Autodesk Fusion 360 part; units mm, degrees
(part 2 of 3)
  spline S18 degree 5 poles (-8.9859, 5.2547) (-8.9893, 5.2567) (-8.9962, 5.2606) (-9.0067, 5.2662) (-9.0209, 5.2733) (-9.0389, 5.2815) (-9.0573, 5.2892) (-9.0757, 5.2967) (-9.0943, 5.304) (-9.1129, 5.3112) (-9.1316, 5.3183) (-9.1504, 5.3252) (-9.1692, 5.332) (-9.1882, 5.3385) (-9.2073, 5.3449) (-9.2265, 5.351) (-9.2458, 5.3569) (-9.2651, 5.3627) (-9.2846, 5.3684) (-9.3041, 5.3739) (-9.3236, 5.3793) (-9.3432, 5.3846) (-9.3629, 5.3898) (-9.3827, 5.3948) (-9.4025, 5.3997) (-9.4224, 5.4044) (-9.4423, 5.409) (-9.4623, 5.4135) (-9.4824, 5.4179) (-9.5025, 5.4221) (-9.5226, 5.4263) (-9.5429, 5.4303) (-9.5631, 5.4342) (-9.5835, 5.438) (-9.6038, 5.4417) (-9.6242, 5.4453) (-9.6447, 5.4488) (-9.6652, 5.4521) (-9.6858, 5.4554) (-9.7064, 5.4585) (-9.7271, 5.4616) (-9.7478, 5.4645) (-9.7685, 5.4674) (-9.7893, 5.4701) (-9.8101, 5.4727) (-9.831, 5.4753) (-9.8519, 5.4777) (-9.8729, 5.4801) (-9.8939, 5.4823) (-9.9149, 5.4844) (-9.936, 5.4865) (-9.9571, 5.4884) (-9.9783, 5.4903) (-9.9994, 5.4921) (-10.0207, 5.4937) (-10.0419, 5.4953) (-10.0632, 5.4968) (-10.0845, 5.4982) (-10.1059, 5.4995) (-10.1273, 5.5007) (-10.1487, 5.5018) (-10.1702, 5.5028) (-10.1917, 5.5037) (-10.2132, 5.5046) (-10.2348, 5.5053) (-10.2564, 5.506) (-10.278, 5.5066) (-10.2997, 5.507) (-10.3213, 5.5074) (-10.3431, 5.5078) (-10.3648, 5.508) (-10.3822, 5.5081) (-10.3953, 5.5081) (-10.404, 5.5081) (-10.4084, 5.5081) knots 0 0 0 0 0 0 0.01428571 0.02857143 0.04285714 0.05714286 0.07142857 0.08571429 0.1 0.11428571 0.12857143 0.14285714 0.15714286 0.17142857 0.18571429 0.2 0.21428571 0.22857143 0.24285714 0.25714286 0.27142857 0.28571429 0.3 0.31428571 0.32857143 0.34285714 0.35714286 0.37142857 0.38571429 0.4 0.41428571 0.42857143 0.44285714 0.45714286 0.47142857 0.48571429 0.5 0.51428571 0.52857143 0.54285714 0.55714286 0.57142857 0.58571429 0.6 0.61428571 0.62857143 0.64285714 0.65714286 0.67142857 0.68571429 0.7 0.71428571 0.72857143 0.74285714 0.75714286 0.77142857 0.78571429 0.8 0.81428571 0.82857143 0.84285714 0.85714286 0.87142857 0.88571429 0.9 0.91428571 0.92857143 0.94285714 0.95714286 0.97142857 0.98571429 1 1 1 1 1 1
  arc A38 (-10.4084, 5.5081) -> (-10.796, 4.7033) centre (0, 0) ccw
  spline S19 degree 5 poles (-10.796, 4.7033) (-10.7932, 4.6999) (-10.7878, 4.6931) (-10.7796, 4.6829) (-10.7687, 4.6694) (-10.7549, 4.6525) (-10.7411, 4.6357) (-10.7273, 4.619) (-10.7134, 4.6024) (-10.6995, 4.5858) (-10.6855, 4.5694) (-10.6715, 4.553) (-10.6574, 4.5367) (-10.6433, 4.5204) (-10.6291, 4.5043) (-10.6149, 4.4882) (-10.6006, 4.4723) (-10.5863, 4.4564) (-10.5719, 4.4405) (-10.5574, 4.4248) (-10.543, 4.4092) (-10.5284, 4.3936) (-10.5138, 4.3782) (-10.4992, 4.3628) (-10.4845, 4.3475) (-10.4698, 4.3323) (-10.455, 4.3172) (-10.4401, 4.3022) (-10.4252, 4.2873) (-10.4103, 4.2724) (-10.3953, 4.2577) (-10.3802, 4.243) (-10.3651, 4.2285) (-10.35, 4.214) (-10.3348, 4.1997) (-10.3195, 4.1854) (-10.3042, 4.1713) (-10.2888, 4.1572) (-10.2734, 4.1433) (-10.2579, 4.1295) (-10.2424, 4.1157) (-10.2268, 4.1021) (-10.2112, 4.0886) (-10.1955, 4.0752) (-10.1797, 4.0619) (-10.1639, 4.0487) (-10.148, 4.0356) (-10.1321, 4.0227) (-10.1161, 4.0098) (-10.1001, 3.9971) (-10.084, 3.9845) (-10.0678, 3.9721) (-10.0516, 3.9597) (-10.0353, 3.9476) (-10.0189, 3.9355) (-10.0025, 3.9236) (-9.986, 3.9118) (-9.9694, 3.9002) (-9.9529, 3.8886) (-9.9362, 3.8773) (-9.9194, 3.8661) (-9.9026, 3.8551) (-9.8856, 3.8444) (-9.8686, 3.8338) (-9.8514, 3.8235) (-9.8342, 3.8133) (-9.817, 3.8032) (-9.7997, 3.7933) (-9.7824, 3.7835) (-9.7649, 3.774) (-9.7472, 3.765) (-9.7329, 3.7583) (-9.7219, 3.7536) (-9.7146, 3.7507) (-9.7109, 3.7492) knots -1 -1 -1 -1 -1 -1 -0.98571429 -0.97142857 -0.95714286 -0.94285714 -0.92857143 -0.91428571 -0.9 -0.88571429 -0.87142857 -0.85714286 -0.84285714 -0.82857143 -0.81428571 -0.8 -0.78571429 -0.77142857 -0.75714286 -0.74285714 -0.72857143 -0.71428571 -0.7 -0.68571429 -0.67142857 -0.65714286 -0.64285714 -0.62857143 -0.61428571 -0.6 -0.58571429 -0.57142857 -0.55714286 -0.54285714 -0.52857143 -0.51428571 -0.5 -0.48571429 -0.47142857 -0.45714286 -0.44285714 -0.42857143 -0.41428571 -0.4 -0.38571429 -0.37142857 -0.35714286 -0.34285714 -0.32857143 -0.31428571 -0.3 -0.28571429 -0.27142857 -0.25714286 -0.24285714 -0.22857143 -0.21428571 -0.2 -0.18571429 -0.17142857 -0.15714286 -0.14285714 -0.12857143 -0.11428571 -0.1 -0.08571429 -0.07142857 -0.05714286 -0.04285714 -0.02857143 -0.01428571 0 0 0 0 0 0
  line L19 (-9.7109, 3.7492) -> (-9.3969, 3.6277)
  arc A39 (-9.0296, 2.8622) -> (-9.3969, 3.6277) centre (-9.6207, 3.0495) ccw
  arc A40 (-9.0296, 2.8622) -> (-9.0729, 2.7218) centre (0, 0) ccw
  arc A41 (-9.8076, 2.2961) -> (-9.0729, 2.7218) centre (-9.6668, 2.8999) ccw
  line L20 (-9.8076, 2.2961) -> (-10.1355, 2.3726)
  spline S20 degree 5 poles (-10.1355, 2.3726) (-10.1394, 2.3735) (-10.1471, 2.3752) (-10.1588, 2.3775) (-10.1744, 2.38) (-10.1941, 2.3826) (-10.2139, 2.3846) (-10.2337, 2.3862) (-10.2536, 2.3877) (-10.2736, 2.3891) (-10.2935, 2.3904) (-10.3135, 2.3915) (-10.3335, 2.3924) (-10.3536, 2.3931) (-10.3737, 2.3935) (-10.3938, 2.3937) (-10.414, 2.3937) (-10.4342, 2.3935) (-10.4544, 2.3932) (-10.4747, 2.3927) (-10.495, 2.3922) (-10.5153, 2.3914) (-10.5356, 2.3905) (-10.5559, 2.3895) (-10.5763, 2.3883) (-10.5967, 2.387) (-10.6171, 2.3855) (-10.6376, 2.3839) (-10.658, 2.3822) (-10.6785, 2.3803) (-10.699, 2.3784) (-10.7195, 2.3762) (-10.74, 2.374) (-10.7606, 2.3717) (-10.7811, 2.3692) (-10.8017, 2.3666) (-10.8223, 2.3639) (-10.8429, 2.361) (-10.8635, 2.3581) (-10.8841, 2.355) (-10.9048, 2.3518) (-10.9254, 2.3485) (-10.9461, 2.3451) (-10.9667, 2.3416) (-10.9874, 2.338) (-11.0081, 2.3343) (-11.0288, 2.3304) (-11.0495, 2.3265) (-11.0703, 2.3225) (-11.091, 2.3183) (-11.1117, 2.3141) (-11.1325, 2.3097) (-11.1532, 2.3052) (-11.174, 2.3007) (-11.1948, 2.296) (-11.2156, 2.2913) (-11.2363, 2.2864) (-11.2571, 2.2814) (-11.2779, 2.2764) (-11.2987, 2.2712) (-11.3195, 2.266) (-11.3403, 2.2606) (-11.3612, 2.2552) (-11.382, 2.2496) (-11.4028, 2.244) (-11.4236, 2.2382) (-11.4445, 2.2324) (-11.4653, 2.2265) (-11.4861, 2.2205) (-11.507, 2.2144) (-11.5278, 2.2082) (-11.5445, 2.2032) (-11.557, 2.1993) (-11.5654, 2.1968) (-11.5695, 2.1955) knots 0 0 0 0 0 0 0.01428571 0.02857143 0.04285714 0.05714286 0.07142857 0.08571429 0.1 0.11428571 0.12857143 0.14285714 0.15714286 0.17142857 0.18571429 0.2 0.21428571 0.22857143 0.24285714 0.25714286 0.27142857 0.28571429 0.3 0.31428571 0.32857143 0.34285714 0.35714286 0.37142857 0.38571429 0.4 0.41428571 0.42857143 0.44285714 0.45714286 0.47142857 0.48571429 0.5 0.51428571 0.52857143 0.54285714 0.55714286 0.57142857 0.58571429 0.6 0.61428571 0.62857143 0.64285714 0.65714286 0.67142857 0.68571429 0.7 0.71428571 0.72857143 0.74285714 0.75714286 0.77142857 0.78571429 0.8 0.81428571 0.82857143 0.84285714 0.85714286 0.87142857 0.88571429 0.9 0.91428571 0.92857143 0.94285714 0.95714286 0.97142857 0.98571429 1 1 1 1 1 1
  arc A42 (-11.5695, 2.1955) -> (-11.7027, 1.3122) centre (0, 0) ccw
  spline S21 degree 5 poles (-11.7027, 1.3122) (-11.6991, 1.3098) (-11.6918, 1.3049) (-11.681, 1.2975) (-11.6666, 1.2878) (-11.6485, 1.2757) (-11.6304, 1.2638) (-11.6122, 1.2519) (-11.594, 1.2401) (-11.5759, 1.2284) (-11.5576, 1.2168) (-11.5394, 1.2052) (-11.5211, 1.1938) (-11.5029, 1.1824) (-11.4845, 1.1712) (-11.4662, 1.16) (-11.4479, 1.149) (-11.4295, 1.138) (-11.4111, 1.1272) (-11.3926, 1.1164) (-11.3742, 1.1057) (-11.3557, 1.0951) (-11.3372, 1.0847) (-11.3187, 1.0743) (-11.3002, 1.064) (-11.2816, 1.0538) (-11.263, 1.0437) (-11.2444, 1.0338) (-11.2258, 1.0239) (-11.2071, 1.0141) (-11.1884, 1.0045) (-11.1697, 0.9949) (-11.151, 0.9855) (-11.1323, 0.9761) (-11.1135, 0.9669) (-11.0947, 0.9578) (-11.0759, 0.9488) (-11.0571, 0.9399) (-11.0382, 0.9311) (-11.0194, 0.9224) (-11.0005, 0.9139) (-10.9816, 0.9054) (-10.9626, 0.8971) (-10.9437, 0.889) (-10.9247, 0.8809) (-10.9057, 0.873) (-10.8867, 0.8652) (-10.8677, 0.8575) (-10.8486, 0.8499) (-10.8295, 0.8425) (-10.8104, 0.8352) (-10.7913, 0.8281) (-10.7722, 0.8211) (-10.753, 0.8142) (-10.7338, 0.8076) (-10.7146, 0.801) (-10.6954, 0.7946) (-10.6761, 0.7884) (-10.6569, 0.7822) (-10.6376, 0.7763) (-10.6183, 0.7705) (-10.5989, 0.765) (-10.5796, 0.7597) (-10.5602, 0.7547) (-10.5408, 0.7499) (-10.5213, 0.7452) (-10.5019, 0.7407) (-10.4824, 0.7362) (-10.463, 0.732) (-10.4435, 0.7281) (-10.4239, 0.7247) (-10.4082, 0.7225) (-10.3964, 0.7213) (-10.3885, 0.7206) (-10.3846, 0.7203) knots -1 -1 -1 -1 -1 -1 -0.98571429 -0.97142857 -0.95714286 -0.94285714 -0.92857143 -0.91428571 -0.9 -0.88571429 -0.87142857 -0.85714286 -0.84285714 -0.82857143 -0.81428571 -0.8 -0.78571429 -0.77142857 -0.75714286 -0.74285714 -0.72857143 -0.71428571 -0.7 -0.68571429 -0.67142857 -0.65714286 -0.64285714 -0.62857143 -0.61428571 -0.6 -0.58571429 -0.57142857 -0.55714286 -0.54285714 -0.52857143 -0.51428571 -0.5 -0.48571429 -0.47142857 -0.45714286 -0.44285714 -0.42857143 -0.41428571 -0.4 -0.38571429 -0.37142857 -0.35714286 -0.34285714 -0.32857143 -0.31428571 -0.3 -0.28571429 -0.27142857 -0.25714286 -0.24285714 -0.22857143 -0.21428571 -0.2 -0.18571429 -0.17142857 -0.15714286 -0.14285714 -0.12857143 -0.11428571 -0.1 -0.08571429 -0.07142857 -0.05714286 -0.04285714 -0.02857143 -0.01428571 0 0 0 0 0 0
  line L21 (-10.3846, 0.7203) -> (-10.0487, 0.6968)
  arc A43 (-9.4721, 0.0735) -> (-10.0487, 0.6968) centre (-10.0921, 0.0783) ccw
  arc A44 (-9.4721, 0.0735) -> (-9.4721, -0.0735) centre (0, 0) ccw
  arc A45 (-10.0487, -0.6968) -> (-9.4721, -0.0735) centre (-10.0921, -0.0783) ccw
  line L22 (-10.0487, -0.6968) -> (-10.3846, -0.7203)
  spline S22 degree 5 poles (-10.3846, -0.7203) (-10.3885, -0.7206) (-10.3964, -0.7213) (-10.4082, -0.7225) (-10.4239, -0.7247) (-10.4435, -0.7281) (-10.463, -0.732) (-10.4824, -0.7362) (-10.5019, -0.7407) (-10.5213, -0.7452) (-10.5408, -0.7499) (-10.5602, -0.7547) (-10.5796, -0.7597) (-10.5989, -0.765) (-10.6183, -0.7705) (-10.6376, -0.7763) (-10.6569, -0.7822) (-10.6761, -0.7884) (-10.6954, -0.7946) (-10.7146, -0.801) (-10.7338, -0.8076) (-10.753, -0.8142) (-10.7722, -0.8211) (-10.7913, -0.8281) (-10.8104, -0.8352) (-10.8295, -0.8425) (-10.8486, -0.8499) (-10.8677, -0.8575) (-10.8867, -0.8652) (-10.9057, -0.873) (-10.9247, -0.8809) (-10.9437, -0.889) (-10.9626, -0.8971) (-10.9816, -0.9054) (-11.0005, -0.9139) (-11.0194, -0.9224) (-11.0382, -0.9311) (-11.0571, -0.9399) (-11.0759, -0.9488) (-11.0947, -0.9578) (-11.1135, -0.9669) (-11.1323, -0.9761) (-11.151, -0.9855) (-11.1697, -0.9949) (-11.1884, -1.0045) (-11.2071, -1.0141) (-11.2258, -1.0239) (-11.2444, -1.0338) (-11.263, -1.0437) (-11.2816, -1.0538) (-11.3002, -1.064) (-11.3187, -1.0743) (-11.3372, -1.0847) (-11.3557, -1.0951) (-11.3742, -1.1057) (-11.3926, -1.1164) (-11.4111, -1.1272) (-11.4295, -1.138) (-11.4479, -1.149) (-11.4662, -1.16) (-11.4845, -1.1712) (-11.5029, -1.1824) (-11.5211, -1.1938) (-11.5394, -1.2052) (-11.5576, -1.2168) (-11.5759, -1.2284) (-11.594, -1.2401) (-11.6122, -1.2519) (-11.6304, -1.2638) (-11.6485, -1.2757) (-11.6666, -1.2878) (-11.681, -1.2975) (-11.6918, -1.3049) (-11.6991, -1.3098) (-11.7027, -1.3122) knots 0 0 0 0 0 0 0.01428571 0.02857143 0.04285714 0.05714286 0.07142857 0.08571429 0.1 0.11428571 0.12857143 0.14285714 0.15714286 0.17142857 0.18571429 0.2 0.21428571 0.22857143 0.24285714 0.25714286 0.27142857 0.28571429 0.3 0.31428571 0.32857143 0.34285714 0.35714286 0.37142857 0.38571429 0.4 0.41428571 0.42857143 0.44285714 0.45714286 0.47142857 0.48571429 0.5 0.51428571 0.52857143 0.54285714 0.55714286 0.57142857 0.58571429 0.6 0.61428571 0.62857143 0.64285714 0.65714286 0.67142857 0.68571429 0.7 0.71428571 0.72857143 0.74285714 0.75714286 0.77142857 0.78571429 0.8 0.81428571 0.82857143 0.84285714 0.85714286 0.87142857 0.88571429 0.9 0.91428571 0.92857143 0.94285714 0.95714286 0.97142857 0.98571429 1 1 1 1 1 1
  arc A46 (-11.7027, -1.3122) -> (-11.5695, -2.1955) centre (0, 0) ccw
  spline S23 degree 5 poles (-11.5695, -2.1955) (-11.5654, -2.1968) (-11.557, -2.1993) (-11.5445, -2.2032) (-11.5278, -2.2082) (-11.507, -2.2144) (-11.4861, -2.2205) (-11.4653, -2.2265) (-11.4445, -2.2324) (-11.4236, -2.2382) (-11.4028, -2.244) (-11.382, -2.2496) (-11.3612, -2.2552) (-11.3403, -2.2606) (-11.3195, -2.266) (-11.2987, -2.2712) (-11.2779, -2.2764) (-11.2571, -2.2814) (-11.2363, -2.2864) (-11.2156, -2.2913) (-11.1948, -2.296) (-11.174, -2.3007) (-11.1532, -2.3052) (-11.1325, -2.3097) (-11.1117, -2.3141) (-11.091, -2.3183) (-11.0703, -2.3225) (-11.0495, -2.3265) (-11.0288, -2.3304) (-11.0081, -2.3343) (-10.9874, -2.338) (-10.9667, -2.3416) (-10.9461, -2.3451) (-10.9254, -2.3485) (-10.9048, -2.3518) (-10.8841, -2.355) (-10.8635, -2.3581) (-10.8429, -2.361) (-10.8223, -2.3639) (-10.8017, -2.3666) (-10.7811, -2.3692) (-10.7606, -2.3717) (-10.74, -2.374) (-10.7195, -2.3762) (-10.699, -2.3784) (-10.6785, -2.3803) (-10.658, -2.3822) (-10.6376, -2.3839) (-10.6171, -2.3855) (-10.5967, -2.387) (-10.5763, -2.3883) (-10.5559, -2.3895) (-10.5356, -2.3905) (-10.5153, -2.3914) (-10.495, -2.3922) (-10.4747, -2.3927) (-10.4544, -2.3932) (-10.4342, -2.3935) (-10.414, -2.3937) (-10.3938, -2.3937) (-10.3737, -2.3935) (-10.3536, -2.3931) (-10.3335, -2.3924) (-10.3135, -2.3915) (-10.2935, -2.3904) (-10.2736, -2.3891) (-10.2536, -2.3877) (-10.2337, -2.3862) (-10.2139, -2.3846) (-10.1941, -2.3826) (-10.1744, -2.38) (-10.1588, -2.3775) (-10.1471, -2.3752) (-10.1394, -2.3735) (-10.1355, -2.3726) knots -1 -1 -1 -1 -1 -1 -0.98571429 -0.97142857 -0.95714286 -0.94285714 -0.92857143 -0.91428571 -0.9 -0.88571429 -0.87142857 -0.85714286 -0.84285714 -0.82857143 -0.81428571 -0.8 -0.78571429 -0.77142857 -0.75714286 -0.74285714 -0.72857143 -0.71428571 -0.7 -0.68571429 -0.67142857 -0.65714286 -0.64285714 -0.62857143 -0.61428571 -0.6 -0.58571429 -0.57142857 -0.55714286 -0.54285714 -0.52857143 -0.51428571 -0.5 -0.48571429 -0.47142857 -0.45714286 -0.44285714 -0.42857143 -0.41428571 -0.4 -0.38571429 -0.37142857 -0.35714286 -0.34285714 -0.32857143 -0.31428571 -0.3 -0.28571429 -0.27142857 -0.25714286 -0.24285714 -0.22857143 -0.21428571 -0.2 -0.18571429 -0.17142857 -0.15714286 -0.14285714 -0.12857143 -0.11428571 -0.1 -0.08571429 -0.07142857 -0.05714286 -0.04285714 -0.02857143 -0.01428571 0 0 0 0 0 0
  line L23 (-10.1355, -2.3726) -> (-9.8076, -2.2961)
  arc A47 (-9.0729, -2.7218) -> (-9.8076, -2.2961) centre (-9.6668, -2.8999) ccw
  arc A48 (-9.0729, -2.7218) -> (-9.0296, -2.8622) centre (0, 0) ccw
  arc A49 (-9.3969, -3.6277) -> (-9.0296, -2.8622) centre (-9.6207, -3.0495) ccw
  line L24 (-9.3969, -3.6277) -> (-9.7109, -3.7492)
  spline S24 degree 5 poles (-9.7109, -3.7492) (-9.7146, -3.7507) (-9.7219, -3.7536) (-9.7329, -3.7583) (-9.7472, -3.765) (-9.7649, -3.774) (-9.7824, -3.7835) (-9.7997, -3.7933) (-9.817, -3.8032) (-9.8342, -3.8133) (-9.8514, -3.8235) (-9.8686, -3.8338) (-9.8856, -3.8444) (-9.9026, -3.8551) (-9.9194, -3.8661) (-9.9362, -3.8773) (-9.9529, -3.8886) (-9.9694, -3.9002) (-9.986, -3.9118) (-10.0025, -3.9236) (-10.0189, -3.9355) (-10.0353, -3.9476) (-10.0516, -3.9597) (-10.0678, -3.9721) (-10.084, -3.9845) (-10.1001, -3.9971) (-10.1161, -4.0098) (-10.1321, -4.0227) (-10.148, -4.0356) (-10.1639, -4.0487) (-10.1797, -4.0619) (-10.1955, -4.0752) (-10.2112, -4.0886) (-10.2268, -4.1021) (-10.2424, -4.1157) (-10.2579, -4.1295) (-10.2734, -4.1433) (-10.2888, -4.1572) (-10.3042, -4.1713) (-10.3195, -4.1854) (-10.3348, -4.1997) (-10.35, -4.214) (-10.3651, -4.2285) (-10.3802, -4.243) (-10.3953, -4.2577) (-10.4103, -4.2724) (-10.4252, -4.2873) (-10.4401, -4.3022) (-10.455, -4.3172) (-10.4698, -4.3323) (-10.4845, -4.3475) (-10.4992, -4.3628) (-10.5138, -4.3782) (-10.5284, -4.3936) (-10.543, -4.4092) (-10.5574, -4.4248) (-10.5719, -4.4405) (-10.5863, -4.4564) (-10.6006, -4.4723) (-10.6149, -4.4882) (-10.6291, -4.5043) (-10.6433, -4.5204) (-10.6574, -4.5367) (-10.6715, -4.553) (-10.6855, -4.5694) (-10.6995, -4.5858) (-10.7134, -4.6024) (-10.7273, -4.619) (-10.7411, -4.6357) (-10.7549, -4.6525) (-10.7687, -4.6694) (-10.7796, -4.6829) (-10.7878, -4.6931) (-10.7932, -4.6999) (-10.796, -4.7033) knots 0 0 0 0 0 0 0.01428571 0.02857143 0.04285714 0.05714286 0.07142857 0.08571429 0.1 0.11428571 0.12857143 0.14285714 0.15714286 0.17142857 0.18571429 0.2 0.21428571 0.22857143 0.24285714 0.25714286 0.27142857 0.28571429 0.3 0.31428571 0.32857143 0.34285714 0.35714286 0.37142857 0.38571429 0.4 0.41428571 0.42857143 0.44285714 0.45714286 0.47142857 0.48571429 0.5 0.51428571 0.52857143 0.54285714 0.55714286 0.57142857 0.58571429 0.6 0.61428571 0.62857143 0.64285714 0.65714286 0.67142857 0.68571429 0.7 0.71428571 0.72857143 0.74285714 0.75714286 0.77142857 0.78571429 0.8 0.81428571 0.82857143 0.84285714 0.85714286 0.87142857 0.88571429 0.9 0.91428571 0.92857143 0.94285714 0.95714286 0.97142857 0.98571429 1 1 1 1 1 1
  arc A50 (-10.796, -4.7033) -> (-10.4084, -5.5081) centre (0, 0) ccw
  spline S25 degree 5 poles (-10.4084, -5.5081) (-10.404, -5.5081) (-10.3953, -5.5081) (-10.3822, -5.5081) (-10.3648, -5.508) (-10.3431, -5.5078) (-10.3213, -5.5074) (-10.2997, -5.507) (-10.278, -5.5066) (-10.2564, -5.506) (-10.2348, -5.5053) (-10.2132, -5.5046) (-10.1917, -5.5037) (-10.1702, -5.5028) (-10.1487, -5.5018) (-10.1273, -5.5007) (-10.1059, -5.4995) (-10.0845, -5.4982) (-10.0632, -5.4968) (-10.0419, -5.4953) (-10.0207, -5.4937) (-9.9994, -5.4921) (-9.9783, -5.4903) (-9.9571, -5.4884) (-9.936, -5.4865) (-9.9149, -5.4844) (-9.8939, -5.4823) (-9.8729, -5.4801) (-9.8519, -5.4777) (-9.831, -5.4753) (-9.8101, -5.4727) (-9.7893, -5.4701) (-9.7685, -5.4674) (-9.7478, -5.4645) (-9.7271, -5.4616) (-9.7064, -5.4585) (-9.6858, -5.4554) (-9.6652, -5.4521) (-9.6447, -5.4488) (-9.6242, -5.4453) (-9.6038, -5.4417) (-9.5835, -5.438) (-9.5631, -5.4342) (-9.5429, -5.4303) (-9.5226, -5.4263) (-9.5025, -5.4221) (-9.4824, -5.4179) (-9.4623, -5.4135) (-9.4423, -5.409) (-9.4224, -5.4044) (-9.4025, -5.3997) (-9.3827, -5.3948) (-9.3629, -5.3898) (-9.3432, -5.3846) (-9.3236, -5.3793) (-9.3041, -5.3739) (-9.2846, -5.3684) (-9.2651, -5.3627) (-9.2458, -5.3569) (-9.2265, -5.351) (-9.2073, -5.3449) (-9.1882, -5.3385) (-9.1692, -5.332) (-9.1504, -5.3252) (-9.1316, -5.3183) (-9.1129, -5.3112) (-9.0943, -5.304) (-9.0757, -5.2967) (-9.0573, -5.2892) (-9.0389, -5.2815) (-9.0209, -5.2733) (-9.0067, -5.2662) (-8.9962, -5.2606) (-8.9893, -5.2567) (-8.9859, -5.2547) knots -1 -1 -1 -1 -1 -1 -0.98571429 -0.97142857 -0.95714286 -0.94285714 -0.92857143 -0.91428571 -0.9 -0.88571429 -0.87142857 -0.85714286 -0.84285714 -0.82857143 -0.81428571 -0.8 -0.78571429 -0.77142857 -0.75714286 -0.74285714 -0.72857143 -0.71428571 -0.7 -0.68571429 -0.67142857 -0.65714286 -0.64285714 -0.62857143 -0.61428571 -0.6 -0.58571429 -0.57142857 -0.55714286 -0.54285714 -0.52857143 -0.51428571 -0.5 -0.48571429 -0.47142857 -0.45714286 -0.44285714 -0.42857143 -0.41428571 -0.4 -0.38571429 -0.37142857 -0.35714286 -0.34285714 -0.32857143 -0.31428571 -0.3 -0.28571429 -0.27142857 -0.25714286 -0.24285714 -0.22857143 -0.21428571 -0.2 -0.18571429 -0.17142857 -0.15714286 -0.14285714 -0.12857143 -0.11428571 -0.1 -0.08571429 -0.07142857 -0.05714286 -0.04285714 -0.02857143 -0.01428571 0 0 0 0 0 0
  line L25 (-8.9859, -5.2547) -> (-8.6951, -5.0849)
  arc A51 (-7.8676, -5.2751) -> (-8.6951, -5.0849) centre (-8.3826, -5.6204) ccw
  arc A52 (-7.8676, -5.2751) -> (-7.7848, -5.3965) centre (0, 0) ccw
  arc A53 (-7.9101, -6.2363) -> (-7.7848, -5.3965) centre (-8.2944, -5.7498) ccw
  line L26 (-7.9101, -6.2363) -> (-8.1744, -6.445)
  spline S26 degree 5 poles (-8.1744, -6.445) (-8.1775, -6.4475) (-8.1836, -6.4524) (-8.1927, -6.4601) (-8.2045, -6.4708) (-8.2187, -6.4846) (-8.2326, -6.4988) (-8.2463, -6.5133) (-8.2598, -6.5279) (-8.2733, -6.5426) (-8.2868, -6.5574) (-8.3001, -6.5723) (-8.3133, -6.5874) (-8.3263, -6.6027) (-8.3392, -6.6181) (-8.3519, -6.6338) (-8.3645, -6.6495) (-8.3769, -6.6654) (-8.3893, -6.6815) (-8.4016, -6.6976) (-8.4138, -6.7138) (-8.4259, -6.7301) (-8.4378, -6.7466) (-8.4497, -6.7631) (-8.4615, -6.7798) (-8.4732, -6.7966) (-8.4848, -6.8135) (-8.4962, -6.8304) (-8.5076, -6.8475) (-8.519, -6.8647) (-8.5302, -6.8819) (-8.5413, -6.8993) (-8.5524, -6.9167) (-8.5633, -6.9342) (-8.5742, -6.9519) (-8.585, -6.9696) (-8.5957, -6.9874) (-8.6063, -7.0052) (-8.6169, -7.0232) (-8.6274, -7.0412) (-8.6377, -7.0593) (-8.648, -7.0775) (-8.6583, -7.0958) (-8.6684, -7.1142) (-8.6785, -7.1326) (-8.6885, -7.1511) (-8.6984, -7.1697) (-8.7082, -7.1883) (-8.718, -7.207) (-8.7277, -7.2258) (-8.7373, -7.2447) (-8.7468, -7.2637) (-8.7562, -7.2827) (-8.7656, -7.3017) (-8.7749, -7.3209) (-8.7842, -7.3401) (-8.7933, -7.3594) (-8.8024, -7.3787) (-8.8114, -7.3981) (-8.8203, -7.4176) (-8.8292, -7.4372) (-8.838, -7.4568) (-8.8467, -7.4764) (-8.8554, -7.4962) (-8.864, -7.516) (-8.8725, -7.5358) (-8.8809, -7.5558) (-8.8893, -7.5757) (-8.8975, -7.5958) (-8.9058, -7.6159) (-8.9139, -7.636) (-8.9204, -7.6522) (-8.9252, -7.6644) (-8.9284, -7.6725) (-8.93, -7.6766) knots 0 0 0 0 0 0 0.01428571 0.02857143 0.04285714 0.05714286 0.07142857 0.08571429 0.1 0.11428571 0.12857143 0.14285714 0.15714286 0.17142857 0.18571429 0.2 0.21428571 0.22857143 0.24285714 0.25714286 0.27142857 0.28571429 0.3 0.31428571 0.32857143 0.34285714 0.35714286 0.37142857 0.38571429 0.4 0.41428571 0.42857143 0.44285714 0.45714286 0.47142857 0.48571429 0.5 0.51428571 0.52857143 0.54285714 0.55714286 0.57142857 0.58571429 0.6 0.61428571 0.62857143 0.64285714 0.65714286 0.67142857 0.68571429 0.7 0.71428571 0.72857143 0.74285714 0.75714286 0.77142857 0.78571429 0.8 0.81428571 0.82857143 0.84285714 0.85714286 0.87142857 0.88571429 0.9 0.91428571 0.92857143 0.94285714 0.95714286 0.97142857 0.98571429 1 1 1 1 1 1
  arc A54 (-8.93, -7.6766) -> (-8.3224, -8.3313) centre (0, 0) ccw
  spline S27 degree 5 poles (-8.3224, -8.3313) (-8.3183, -8.3301) (-8.3099, -8.3275) (-8.2974, -8.3236) (-8.2808, -8.3183) (-8.2601, -8.3117) (-8.2395, -8.305) (-8.2188, -8.2983) (-8.1983, -8.2914) (-8.1778, -8.2845) (-8.1574, -8.2775) (-8.137, -8.2704) (-8.1167, -8.2633) (-8.0964, -8.256) (-8.0762, -8.2487) (-8.056, -8.2414) (-8.0359, -8.2339) (-8.0159, -8.2264) (-7.9959, -8.2188) (-7.976, -8.2111) (-7.9562, -8.2033) (-7.9364, -8.1955) (-7.9167, -8.1875) (-7.897, -8.1795) (-7.8774, -8.1714) (-7.8579, -8.1633) (-7.8384, -8.155) (-7.819, -8.1467) (-7.7997, -8.1383) (-7.7804, -8.1298) (-7.7612, -8.1212) (-7.7421, -8.1125) (-7.723, -8.1038) (-7.704, -8.095) (-7.6851, -8.086) (-7.6663, -8.077) (-7.6475, -8.068) (-7.6288, -8.0588) (-7.6102, -8.0495) (-7.5916, -8.0402) (-7.5732, -8.0307) (-7.5548, -8.0212) (-7.5365, -8.0116) (-7.5183, -8.0019) (-7.5002, -7.992) (-7.4821, -7.9821) (-7.4641, -7.9721) (-7.4463, -7.9621) (-7.4285, -7.9519) (-7.4108, -7.9416) (-7.3932, -7.9312) (-7.3757, -7.9207) (-7.3583, -7.9101) (-7.341, -7.8993) (-7.3238, -7.8885) (-7.3067, -7.8776) (-7.2897, -7.8665) (-7.2728, -7.8554) (-7.256, -7.8442) (-7.2393, -7.8328) (-7.2228, -7.8213) (-7.2064, -7.8096) (-7.1902, -7.7978) (-7.1742, -7.7857) (-7.1583, -7.7736) (-7.1426, -7.7613) (-7.1269, -7.7489) (-7.1113, -7.7365) (-7.0958, -7.7239) (-7.0806, -7.7111) (-7.0658, -7.698) (-7.0543, -7.687) (-7.046, -7.6786) (-7.0405, -7.6728) (-7.0379, -7.6699) knots -1 -1 -1 -1 -1 -1 -0.98571429 -0.97142857 -0.95714286 -0.94285714 -0.92857143 -0.91428571 -0.9 -0.88571429 -0.87142857 -0.85714286 -0.84285714 -0.82857143 -0.81428571 -0.8 -0.78571429 -0.77142857 -0.75714286 -0.74285714 -0.72857143 -0.71428571 -0.7 -0.68571429 -0.67142857 -0.65714286 -0.64285714 -0.62857143 -0.61428571 -0.6 -0.58571429 -0.57142857 -0.55714286 -0.54285714 -0.52857143 -0.51428571 -0.5 -0.48571429 -0.47142857 -0.45714286 -0.44285714 -0.42857143 -0.41428571 -0.4 -0.38571429 -0.37142857 -0.35714286 -0.34285714 -0.32857143 -0.31428571 -0.3 -0.28571429 -0.27142857 -0.25714286 -0.24285714 -0.22857143 -0.21428571 -0.2 -0.18571429 -0.17142857 -0.15714286 -0.14285714 -0.12857143 -0.11428571 -0.1 -0.08571429 -0.07142857 -0.05714286 -0.04285714 -0.02857143 -0.01428571 0 0 0 0 0 0
  line L27 (-7.0379, -7.6699) -> (-6.81, -7.422)
  arc A55 (-5.9632, -7.3598) -> (-6.81, -7.422) centre (-6.3535, -7.8415) ccw
  arc A56 (-5.9632, -7.3598) -> (-5.8483, -7.4514) centre (0, 0) ccw
  arc A57 (-5.7205, -8.2908) -> (-5.8483, -7.4514) centre (-6.2311, -7.9391) ccw
  line L28 (-5.7205, -8.2908) -> (-5.9115, -8.5681)
  spline S28 degree 5 poles (-5.9115, -8.5681) (-5.9137, -8.5714) (-5.9182, -8.5779) (-5.9246, -8.588) (-5.9327, -8.6016) (-5.9422, -8.619) (-5.9513, -8.6367) (-5.9601, -8.6545) (-5.9688, -8.6725) (-5.9773, -8.6905) (-5.9858, -8.7086) (-5.9941, -8.7268) (-6.0023, -8.7451) (-6.0102, -8.7636) (-6.018, -8.7821) (-6.0255, -8.8008) (-6.0329, -8.8196) (-6.0401, -8.8385) (-6.0472, -8.8574) (-6.0542, -8.8764) (-6.061, -8.8955) (-6.0678, -8.9147) (-6.0744, -8.9339) (-6.0809, -8.9533) (-6.0872, -8.9727) (-6.0934, -8.9921) (-6.0995, -9.0117) (-6.1055, -9.0313) (-6.1113, -9.051) (-6.1171, -9.0707) (-6.1227, -9.0905) (-6.1283, -9.1104) (-6.1337, -9.1303) (-6.139, -9.1503) (-6.1442, -9.1703) (-6.1493, -9.1904) (-6.1543, -9.2106) (-6.1592, -9.2308) (-6.1639, -9.251) (-6.1686, -9.2714) (-6.1732, -9.2917) (-6.1777, -9.3122) (-6.1821, -9.3326) (-6.1864, -9.3532) (-6.1906, -9.3737) (-6.1946, -9.3944) (-6.1986, -9.415) (-6.2025, -9.4358) (-6.2063, -9.4565) (-6.2101, -9.4773) (-6.2137, -9.4982) (-6.2172, -9.5191) (-6.2206, -9.5401) (-6.224, -9.5611) (-6.2272, -9.5821) (-6.2304, -9.6032) (-6.2334, -9.6243) (-6.2364, -9.6455) (-6.2393, -9.6667) (-6.2421, -9.6879) (-6.2448, -9.7092) (-6.2474, -9.7305) (-6.25, -9.7519) (-6.2524, -9.7733) (-6.2548, -9.7948) (-6.2571, -9.8162) (-6.2592, -9.8378) (-6.2613, -9.8593) (-6.2634, -9.8809) (-6.2653, -9.9025) (-6.2671, -9.9242) (-6.2685, -9.9416) (-6.2696, -9.9546) (-6.2702, -9.9633) (-6.2706, -9.9677) knots 0 0 0 0 0 0 0.01428571 0.02857143 0.04285714 0.05714286 0.07142857 0.08571429 0.1 0.11428571 0.12857143 0.14285714 0.15714286 0.17142857 0.18571429 0.2 0.21428571 0.22857143 0.24285714 0.25714286 0.27142857 0.28571429 0.3 0.31428571 0.32857143 0.34285714 0.35714286 0.37142857 0.38571429 0.4 0.41428571 0.42857143 0.44285714 0.45714286 0.47142857 0.48571429 0.5 0.51428571 0.52857143 0.54285714 0.55714286 0.57142857 0.58571429 0.6 0.61428571 0.62857143 0.64285714 0.65714286 0.67142857 0.68571429 0.7 0.71428571 0.72857143 0.74285714 0.75714286 0.77142857 0.78571429 0.8 0.81428571 0.82857143 0.84285714 0.85714286 0.87142857 0.88571429 0.9 0.91428571 0.92857143 0.94285714 0.95714286 0.97142857 0.98571429 1 1 1 1 1 1
  arc A58 (-6.2706, -9.9677) -> (-5.497, -10.4143) centre (0, 0) ccw
  spline S29 degree 5 poles (-5.497, -10.4143) (-5.4934, -10.4118) (-5.4862, -10.4069) (-5.4754, -10.3995) (-5.4611, -10.3896) (-5.4432, -10.3772) (-5.4254, -10.3647) (-5.4078, -10.3521) (-5.3901, -10.3395) (-5.3726, -10.3269) (-5.3551, -10.3142) (-5.3377, -10.3014) (-5.3204, -10.2886) (-5.3032, -10.2757) (-5.286, -10.2628) (-5.2689, -10.2498) (-5.2519, -10.2367) (-5.235, -10.2236) (-5.2182, -10.2105) (-5.2014, -10.1972) (-5.1847, -10.184) (-5.1681, -10.1706) (-5.1516, -10.1572) (-5.1352, -10.1438) (-5.1189, -10.1303) (-5.1026, -10.1167) (-5.0864, -10.1031) (-5.0703, -10.0894) (-5.0543, -10.0757) (-5.0384, -10.0619) (-5.0226, -10.048) (-5.0069, -10.0341) (-4.9913, -10.0202) (-4.9757, -10.0061) (-4.9603, -9.992) (-4.9449, -9.9779) (-4.9297, -9.9637) (-4.9145, -9.9494) (-4.8994, -9.935) (-4.8845, -9.9206) (-4.8696, -9.9062) (-4.8549, -9.8917) (-4.8402, -9.8771) (-4.8257, -9.8624) (-4.8112, -9.8477) (-4.7969, -9.8329) (-4.7827, -9.8181) (-4.7686, -9.8031) (-4.7546, -9.7882) (-4.7407, -9.7731) (-4.727, -9.758) (-4.7133, -9.7428) (-4.6998, -9.7275) (-4.6865, -9.7122) (-4.6732, -9.6968) (-4.6601, -9.6813) (-4.6472, -9.6657) (-4.6343, -9.6501) (-4.6215, -9.6344) (-4.609, -9.6186) (-4.5966, -9.6028) (-4.5844, -9.5868) (-4.5724, -9.5707) (-4.5606, -9.5545) (-4.549, -9.5382) (-4.5376, -9.5218) (-4.5262, -9.5053) (-4.515, -9.4889) (-4.5039, -9.4723) (-4.4932, -9.4556) (-4.4829, -9.4386) (-4.4751, -9.4248) (-4.4696, -9.4143) (-4.4662, -9.4071) (-4.4645, -9.4036) knots -1 -1 -1 -1 -1 -1 -0.98571429 -0.97142857 -0.95714286 -0.94285714 -0.92857143 -0.91428571 -0.9 -0.88571429 -0.87142857 -0.85714286 -0.84285714 -0.82857143 -0.81428571 -0.8 -0.78571429 -0.77142857 -0.75714286 -0.74285714 -0.72857143 -0.71428571 -0.7 -0.68571429 -0.67142857 -0.65714286 -0.64285714 -0.62857143 -0.61428571 -0.6 -0.58571429 -0.57142857 -0.55714286 -0.54285714 -0.52857143 -0.51428571 -0.5 -0.48571429 -0.47142857 -0.45714286 -0.44285714 -0.42857143 -0.41428571 -0.4 -0.38571429 -0.37142857 -0.35714286 -0.34285714 -0.32857143 -0.31428571 -0.3 -0.28571429 -0.27142857 -0.25714286 -0.24285714 -0.22857143 -0.21428571 -0.2 -0.18571429 -0.17142857 -0.15714286 -0.14285714 -0.12857143 -0.11428571 -0.1 -0.08571429 -0.07142857 -0.05714286 -0.04285714 -0.02857143 -0.01428571 0 0 0 0 0 0
  line L29 (-4.4645, -9.4036) -> (-4.3198, -9.0995)
  arc A59 (-3.5289, -8.7905) -> (-4.3198, -9.0995) centre (-3.7599, -9.3659) ccw
  arc A60 (-3.5289, -8.7905) -> (-3.3922, -8.8442) centre (0, 0) ccw
  arc A61 (-3.0226, -9.6086) -> (-3.3922, -8.8442) centre (-3.6142, -9.4231) ccw
  line L30 (-3.0226, -9.6086) -> (-3.1234, -9.9299)
  spline S30 degree 5 poles (-3.1234, -9.9299) (-3.1246, -9.9337) (-3.1268, -9.9413) (-3.13, -9.9527) (-3.1337, -9.9681) (-3.1377, -9.9876) (-3.1412, -10.0071) (-3.1443, -10.0268) (-3.1473, -10.0465) (-3.1502, -10.0663) (-3.1529, -10.0861) (-3.1555, -10.1059) (-3.1579, -10.1258) (-3.1601, -10.1458) (-3.162, -10.1658) (-3.1637, -10.1859) (-3.1652, -10.206) (-3.1666, -10.2261) (-3.1678, -10.2464) (-3.1688, -10.2666) (-3.1698, -10.2869) (-3.1705, -10.3072) (-3.1712, -10.3275) (-3.1717, -10.3479) (-3.172, -10.3683) (-3.1722, -10.3887) (-3.1723, -10.4092) (-3.1722, -10.4297) (-3.172, -10.4502) (-3.1717, -10.4708) (-3.1712, -10.4913) (-3.1707, -10.512) (-3.17, -10.5326) (-3.1692, -10.5532) (-3.1682, -10.5739) (-3.1672, -10.5946) (-3.166, -10.6154) (-3.1647, -10.6361) (-3.1633, -10.6569) (-3.1618, -10.6777) (-3.1602, -10.6985) (-3.1584, -10.7194) (-3.1566, -10.7402) (-3.1546, -10.7611) (-3.1526, -10.782) (-3.1504, -10.8029) (-3.1481, -10.8238) (-3.1457, -10.8448) (-3.1432, -10.8658) (-3.1407, -10.8867) (-3.138, -10.9077) (-3.1352, -10.9288) (-3.1323, -10.9498) (-3.1293, -10.9708) (-3.1262, -10.9919) (-3.123, -11.013) (-3.1197, -11.0341) (-3.1163, -11.0552) (-3.1128, -11.0763) (-3.1092, -11.0974) (-3.1055, -11.1185) (-3.1018, -11.1397) (-3.0979, -11.1609) (-3.0939, -11.182) (-3.0898, -11.2032) (-3.0857, -11.2244) (-3.0814, -11.2456) (-3.0771, -11.2669) (-3.0726, -11.2881) (-3.0681, -11.3093) (-3.0635, -11.3306) (-3.0597, -11.3476) (-3.0568, -11.3603) (-3.0549, -11.3689) (-3.0539, -11.3731) knots 0 0 0 0 0 0 0.01428571 0.02857143 0.04285714 0.05714286 0.07142857 0.08571429 0.1 0.11428571 0.12857143 0.14285714 0.15714286 0.17142857 0.18571429 0.2 0.21428571 0.22857143 0.24285714 0.25714286 0.27142857 0.28571429 0.3 0.31428571 0.32857143 0.34285714 0.35714286 0.37142857 0.38571429 0.4 0.41428571 0.42857143 0.44285714 0.45714286 0.47142857 0.48571429 0.5 0.51428571 0.52857143 0.54285714 0.55714286 0.57142857 0.58571429 0.6 0.61428571 0.62857143 0.64285714 0.65714286 0.67142857 0.68571429 0.7 0.71428571 0.72857143 0.74285714 0.75714286 0.77142857 0.78571429 0.8 0.81428571 0.82857143 0.84285714 0.85714286 0.87142857 0.88571429 0.9 0.91428571 0.92857143 0.94285714 0.95714286 0.97142857 0.98571429 1 1 1 1 1 1
  arc A62 (-3.0539, -11.3731) -> (-2.1831, -11.5719) centre (0, 0) ccw
  spline S31 degree 5 poles (-2.1831, -11.5719) (-2.1804, -11.5685) (-2.1749, -11.5616) (-2.1668, -11.5514) (-2.156, -11.5377) (-2.1427, -11.5206) (-2.1294, -11.5034) (-2.1162, -11.4862) (-2.103, -11.469) (-2.09, -11.4517) (-2.0771, -11.4344) (-2.0642, -11.4171) (-2.0514, -11.3997) (-2.0388, -11.3823) (-2.0262, -11.3649) (-2.0137, -11.3475) (-2.0013, -11.33) (-1.989, -11.3125) (-1.9768, -11.2949) (-1.9646, -11.2774) (-1.9526, -11.2598) (-1.9407, -11.2421) (-1.9288, -11.2245) (-1.9171, -11.2068) (-1.9055, -11.189) (-1.8939, -11.1713) (-1.8825, -11.1535) (-1.8712, -11.1357) (-1.8599, -11.1179) (-1.8488, -11.1) (-1.8378, -11.0821) (-1.8268, -11.0641) (-1.816, -11.0462) (-1.8053, -11.0282) (-1.7947, -11.0102) (-1.7842, -10.9921) (-1.7738, -10.974) (-1.7635, -10.9559) (-1.7534, -10.9378) (-1.7433, -10.9196) (-1.7334, -10.9014) (-1.7236, -10.8832) (-1.7139, -10.8649) (-1.7043, -10.8466) (-1.6948, -10.8283) (-1.6855, -10.81) (-1.6763, -10.7916) (-1.6672, -10.7732) (-1.6582, -10.7547) (-1.6494, -10.7363) (-1.6407, -10.7178) (-1.6322, -10.6992) (-1.6238, -10.6807) (-1.6155, -10.6621) (-1.6074, -10.6434) (-1.5995, -10.6248) (-1.5917, -10.6061) (-1.584, -10.5874) (-1.5764, -10.5686) (-1.5691, -10.5498) (-1.5619, -10.531) (-1.5549, -10.5121) (-1.5482, -10.4932) (-1.5417, -10.4743) (-1.5355, -10.4553) (-1.5294, -10.4362) (-1.5234, -10.4172) (-1.5175, -10.3981) (-1.5118, -10.379) (-1.5065, -10.3599) (-1.5016, -10.3406) (-1.4983, -10.3251) (-1.4962, -10.3135) (-1.4949, -10.3056) (-1.4944, -10.3017) knots -1 -1 -1 -1 -1 -1 -0.98571429 -0.97142857 -0.95714286 -0.94285714 -0.92857143 -0.91428571 -0.9 -0.88571429 -0.87142857 -0.85714286 -0.84285714 -0.82857143 -0.81428571 -0.8 -0.78571429 -0.77142857 -0.75714286 -0.74285714 -0.72857143 -0.71428571 -0.7 -0.68571429 -0.67142857 -0.65714286 -0.64285714 -0.62857143 -0.61428571 -0.6 -0.58571429 -0.57142857 -0.55714286 -0.54285714 -0.52857143 -0.51428571 -0.5 -0.48571429 -0.47142857 -0.45714286 -0.44285714 -0.42857143 -0.41428571 -0.4 -0.38571429 -0.37142857 -0.35714286 -0.34285714 -0.32857143 -0.31428571 -0.3 -0.28571429 -0.27142857 -0.25714286 -0.24285714 -0.22857143 -0.21428571 -0.2 -0.18571429 -0.17142857 -0.15714286 -0.14285714 -0.12857143 -0.11428571 -0.1 -0.08571429 -0.07142857 -0.05714286 -0.04285714 -0.02857143 -0.01428571 0 0 0 0 0 0
  line L31 (-1.4944, -10.3017) -> (-1.4457, -9.9685)
  arc A63 (-0.7811, -9.4401) -> (-1.4457, -9.9685) centre (-0.8322, -10.058) ccw
  arc A64 (-0.7811, -9.4401) -> (-0.6346, -9.4511) centre (0, 0) ccw
  arc A65 (-0.0561, -10.0726) -> (-0.6346, -9.4511) centre (-0.6761, -10.0697) ccw
  line L32 (-0.0561, -10.0726) -> (-0.0577, -10.4094)
  spline S32 degree 5 poles (-0.0577, -10.4094) (-0.0577, -10.4133) (-0.0577, -10.4213) (-0.0573, -10.4331) (-0.0564, -10.4489) (-0.0544, -10.4687) (-0.052, -10.4884) (-0.0492, -10.5081) (-0.0462, -10.5279) (-0.0431, -10.5476) (-0.0399, -10.5673) (-0.0366, -10.5871) (-0.033, -10.6068) (-0.0292, -10.6265) (-0.0251, -10.6462) (-0.0208, -10.6659) (-0.0163, -10.6855) (-0.0117, -10.7052) (-0.0069, -10.7248) (-0.0019, -10.7445) (0.0032, -10.7641) (0.0084, -10.7838) (0.0138, -10.8034) (0.0193, -10.823) (0.025, -10.8426) (0.0308, -10.8622) (0.0368, -10.8818) (0.0429, -10.9013) (0.0492, -10.9209) (0.0555, -10.9404) (0.062, -10.96) (0.0686, -10.9795) (0.0754, -10.999) (0.0823, -11.0185) (0.0892, -11.038) (0.0964, -11.0575) (0.1036, -11.077) (0.1109, -11.0964) (0.1184, -11.1158) (0.126, -11.1353) (0.1337, -11.1547) (0.1415, -11.1741) (0.1494, -11.1935) (0.1574, -11.2128) (0.1655, -11.2322) (0.1738, -11.2516) (0.1821, -11.2709) (0.1906, -11.2902) (0.1991, -11.3095) (0.2078, -11.3288) (0.2166, -11.3481) (0.2254, -11.3673) (0.2344, -11.3866) (0.2435, -11.4058) (0.2526, -11.425) (0.2619, -11.4442) (0.2713, -11.4634) (0.2807, -11.4826) (0.2903, -11.5017) (0.2999, -11.5208) (0.3097, -11.54) (0.3195, -11.5591) (0.3295, -11.5781) (0.3395, -11.5972) (0.3496, -11.6163) (0.3599, -11.6353) (0.3702, -11.6543) (0.3806, -11.6733) (0.3911, -11.6923) (0.4017, -11.7112) (0.4124, -11.7302) (0.421, -11.7453) (0.4275, -11.7567) (0.4318, -11.7642) (0.434, -11.768) knots 0 0 0 0 0 0 0.01428571 0.02857143 0.04285714 0.05714286 0.07142857 0.08571429 0.1 0.11428571 0.12857143 0.14285714 0.15714286 0.17142857 0.18571429 0.2 0.21428571 0.22857143 0.24285714 0.25714286 0.27142857 0.28571429 0.3 0.31428571 0.32857143 0.34285714 0.35714286 0.37142857 0.38571429 0.4 0.41428571 0.42857143 0.44285714 0.45714286 0.47142857 0.48571429 0.5 0.51428571 0.52857143 0.54285714 0.55714286 0.57142857 0.58571429 0.6 0.61428571 0.62857143 0.64285714 0.65714286 0.67142857 0.68571429 0.7 0.71428571 0.72857143 0.74285714 0.75714286 0.77142857 0.78571429 0.8 0.81428571 0.82857143 0.84285714 0.85714286 0.87142857 0.88571429 0.9 0.91428571 0.92857143 0.94285714 0.95714286 0.97142857 0.98571429 1 1 1 1 1 1
  arc A66 (0.434, -11.768) -> (1.3248, -11.7012) centre (0, 0) ccw
  spline S33 degree 5 poles (1.3248, -11.7012) (1.3264, -11.6972) (1.3295, -11.6891) (1.3343, -11.6769) (1.3405, -11.6606) (1.3483, -11.6403) (1.3559, -11.62) (1.3635, -11.5996) (1.3709, -11.5793) (1.3783, -11.559) (1.3856, -11.5386) (1.3928, -11.5183) (1.3998, -11.4979) (1.4068, -11.4776) (1.4137, -11.4572) (1.4205, -11.4369) (1.4272, -11.4165) (1.4338, -11.3961) (1.4403, -11.3758) (1.4467, -11.3554) (1.453, -11.3351) (1.4592, -11.3147) (1.4653, -11.2943) (1.4713, -11.274) (1.4772, -11.2536) (1.483, -11.2332) (1.4887, -11.2129) (1.4943, -11.1925) (1.4997, -11.1721) (1.5051, -11.1518) (1.5104, -11.1314) (1.5155, -11.1111) (1.5206, -11.0907) (1.5255, -11.0704) (1.5303, -11.05) (1.535, -11.0297) (1.5396, -11.0093) (1.5441, -10.989) (1.5485, -10.9687) (1.5527, -10.9483) (1.5569, -10.928) (1.5609, -10.9077) (1.5648, -10.8874) (1.5685, -10.8671) (1.5722, -10.8468) (1.5757, -10.8265) (1.5791, -10.8063) (1.5823, -10.786) (1.5854, -10.7657) (1.5884, -10.7455) (1.5913, -10.7252) (1.594, -10.705) (1.5965, -10.6848) (1.5989, -10.6646) (1.6012, -10.6444) (1.6033, -10.6242) (1.6052, -10.604) (1.6071, -10.5839) (1.6088, -10.5637) (1.6103, -10.5436) (1.6116, -10.5235) (1.6127, -10.5034) (1.6135, -10.4834) (1.6141, -10.4634) (1.6145, -10.4433) (1.6147, -10.4234) (1.6148, -10.4034) (1.6148, -10.3835) (1.6146, -10.3635) (1.6141, -10.3437) (1.6131, -10.3238) (1.6117, -10.3081) (1.6102, -10.2963) (1.6091, -10.2884) (1.6085, -10.2845) knots -1 -1 -1 -1 -1 -1 -0.98571429 -0.97142857 -0.95714286 -0.94285714 -0.92857143 -0.91428571 -0.9 -0.88571429 -0.87142857 -0.85714286 -0.84285714 -0.82857143 -0.81428571 -0.8 -0.78571429 -0.77142857 -0.75714286 -0.74285714 -0.72857143 -0.71428571 -0.7 -0.68571429 -0.67142857 -0.65714286 -0.64285714 -0.62857143 -0.61428571 -0.6 -0.58571429 -0.57142857 -0.55714286 -0.54285714 -0.52857143 -0.51428571 -0.5 -0.48571429 -0.47142857 -0.45714286 -0.44285714 -0.42857143 -0.41428571 -0.4 -0.38571429 -0.37142857 -0.35714286 -0.34285714 -0.32857143 -0.31428571 -0.3 -0.28571429 -0.27142857 -0.25714286 -0.24285714 -0.22857143 -0.21428571 -0.2 -0.18571429 -0.17142857 -0.15714286 -0.14285714 -0.12857143 -0.11428571 -0.1 -0.08571429 -0.07142857 -0.05714286 -0.04285714 -0.02857143 -0.01428571 0 0 0 0 0 0
  line L33 (1.6085, -10.2845) -> (1.5568, -9.9518)
  arc A67 (2.0361, -9.251) -> (1.5568, -9.9518) centre (2.1694, -9.8565) ccw
  arc A68 (2.0361, -9.251) -> (2.1794, -9.2183) centre (0, 0) ccw
  arc A69 (2.9153, -9.6417) -> (2.1794, -9.2183) centre (2.322, -9.8216) ccw
  line L34 (2.9153, -9.6417) -> (3.0131, -9.9639)
  spline S34 degree 5 poles (3.0131, -9.9639) (3.0142, -9.9677) (3.0166, -9.9753) (3.0204, -9.9865) (3.026, -10.0013) (3.0337, -10.0196) (3.0419, -10.0378) (3.0503, -10.0558) (3.059, -10.0738) (3.0677, -10.0917) (3.0766, -10.1096) (3.0856, -10.1275) (3.0949, -10.1453) (3.1043, -10.163) (3.114, -10.1806) (3.1239, -10.1981) (3.134, -10.2156) (3.1443, -10.233) (3.1546, -10.2504) (3.1652, -10.2677) (3.1758, -10.285) (3.1866, -10.3022) (3.1975, -10.3194) (3.2086, -10.3365) (3.2198, -10.3535) (3.2312, -10.3705) (3.2426, -10.3875) (3.2542, -10.4044) (3.266, -10.4212) (3.2778, -10.438) (3.2898, -10.4548) (3.3019, -10.4715) (3.3141, -10.4881) (3.3264, -10.5048) (3.3388, -10.5213) (3.3513, -10.5378) (3.364, -10.5543) (3.3767, -10.5707) (3.3896, -10.5871) (3.4026, -10.6034) (3.4156, -10.6197) (3.4288, -10.636) (3.4421, -10.6521) (3.4555, -10.6683) (3.4689, -10.6844) (3.4825, -10.7005) (3.4962, -10.7165) (3.51, -10.7324) (3.5238, -10.7484) (3.5378, -10.7642) (3.5518, -10.7801) (3.566, -10.7959) (3.5802, -10.8116) (3.5946, -10.8273) (3.609, -10.843) (3.6235, -10.8586) (3.6381, -10.8742) (3.6528, -10.8897) (3.6676, -10.9052) (3.6824, -10.9206) (3.6974, -10.936) (3.7124, -10.9513) (3.7276, -10.9666) (3.7428, -10.9819) (3.7581, -10.9971) (3.7734, -11.0123) (3.7889, -11.0274) (3.8044, -11.0425) (3.8201, -11.0575) (3.8358, -11.0725) (3.8516, -11.0875) (3.8643, -11.0994) (3.8738, -11.1083) (3.8802, -11.1143) (3.8834, -11.1173) knots 0 0 0 0 0 0 0.01428571 0.02857143 0.04285714 0.05714286 0.07142857 0.08571429 0.1 0.11428571 0.12857143 0.14285714 0.15714286 0.17142857 0.18571429 0.2 0.21428571 0.22857143 0.24285714 0.25714286 0.27142857 0.28571429 0.3 0.31428571 0.32857143 0.34285714 0.35714286 0.37142857 0.38571429 0.4 0.41428571 0.42857143 0.44285714 0.45714286 0.47142857 0.48571429 0.5 0.51428571 0.52857143 0.54285714 0.55714286 0.57142857 0.58571429 0.6 0.61428571 0.62857143 0.64285714 0.65714286 0.67142857 0.68571429 0.7 0.71428571 0.72857143 0.74285714 0.75714286 0.77142857 0.78571429 0.8 0.81428571 0.82857143 0.84285714 0.85714286 0.87142857 0.88571429 0.9 0.91428571 0.92857143 0.94285714 0.95714286 0.97142857 0.98571429 1 1 1 1 1 1
  arc A70 (3.8834, -11.1173) -> (4.7149, -10.7909) centre (0, 0) ccw
  spline S35 degree 5 poles (4.7149, -10.7909) (4.7152, -10.7866) (4.7159, -10.7779) (4.7168, -10.7648) (4.718, -10.7474) (4.7194, -10.7257) (4.7207, -10.7041) (4.722, -10.6824) (4.7231, -10.6608) (4.7241, -10.6392) (4.7251, -10.6176) (4.7259, -10.596) (4.7267, -10.5745) (4.7274, -10.553) (4.728, -10.5315) (4.7285, -10.5101) (4.7289, -10.4886) (4.7292, -10.4672) (4.7294, -10.4459) (4.7295, -10.4245) (4.7295, -10.4032) (4.7294, -10.3819) (4.7293, -10.3606) (4.729, -10.3394) (4.7286, -10.3182) (4.7282, -10.297) (4.7276, -10.2759) (4.7269, -10.2548) (4.7262, -10.2337) (4.7253, -10.2127) (4.7243, -10.1917) (4.7233, -10.1707) (4.7221, -10.1498) (4.7208, -10.1289) (4.7194, -10.108) (4.7179, -10.0872) (4.7163, -10.0664) (4.7146, -10.0457) (4.7128, -10.0249) (4.7108, -10.0043) (4.7088, -9.9836) (4.7066, -9.963) (4.7044, -9.9425) (4.702, -9.922) (4.6995, -9.9015) (4.6968, -9.8811) (4.6941, -9.8607) (4.6912, -9.8404) (4.6883, -9.8201) (4.6851, -9.7999) (4.6819, -9.7797) (4.6785, -9.7596) (4.675, -9.7395) (4.6713, -9.7195) (4.6675, -9.6995) (4.6636, -9.6796) (4.6595, -9.6598) (4.6553, -9.64) (4.651, -9.6202) (4.6465, -9.6006) (4.6418, -9.581) (4.637, -9.5615) (4.6318, -9.542) (4.6265, -9.5227) (4.621, -9.5035) (4.6153, -9.4843) (4.6095, -9.4652) (4.6036, -9.4462) (4.5976, -9.4272) (4.5912, -9.4084) (4.5844, -9.3897) (4.5784, -9.375) (4.5736, -9.3642) (4.5702, -9.357) (4.5685, -9.3535) knots -1 -1 -1 -1 -1 -1 -0.98571429 -0.97142857 -0.95714286 -0.94285714 -0.92857143 -0.91428571 -0.9 -0.88571429 -0.87142857 -0.85714286 -0.84285714 -0.82857143 -0.81428571 -0.8 -0.78571429 -0.77142857 -0.75714286 -0.74285714 -0.72857143 -0.71428571 -0.7 -0.68571429 -0.67142857 -0.65714286 -0.64285714 -0.62857143 -0.61428571 -0.6 -0.58571429 -0.57142857 -0.55714286 -0.54285714 -0.52857143 -0.51428571 -0.5 -0.48571429 -0.47142857 -0.45714286 -0.44285714 -0.42857143 -0.41428571 -0.4 -0.38571429 -0.37142857 -0.35714286 -0.34285714 -0.32857143 -0.31428571 -0.3 -0.28571429 -0.27142857 -0.25714286 -0.24285714 -0.22857143 -0.21428571 -0.2 -0.18571429 -0.17142857 -0.15714286 -0.14285714 -0.12857143 -0.11428571 -0.1 -0.08571429 -0.07142857 -0.05714286 -0.04285714 -0.02857143 -0.01428571 0 0 0 0 0 0
  line L35 (4.5685, -9.3535) -> (4.4209, -9.0508)
  arc A71 (4.6724, -8.2398) -> (4.4209, -9.0508) centre (4.9783, -8.7791) ccw
  arc A72 (4.6724, -8.2398) -> (4.7997, -8.1664) centre (0, 0) ccw
  arc A73 (5.6277, -8.354) -> (4.7997, -8.1664) centre (5.1138, -8.7009) ccw
  line L36 (5.6277, -8.354) -> (5.8161, -8.6331)
  spline S36 degree 5 poles (5.8161, -8.6331) (5.8183, -8.6364) (5.8228, -8.6429) (5.8298, -8.6526) (5.8395, -8.6651) (5.8523, -8.6803) (5.8654, -8.6952) (5.8788, -8.7099) (5.8924, -8.7246) (5.906, -8.7391) (5.9198, -8.7536) (5.9337, -8.768) (5.9477, -8.7823) (5.962, -8.7965) (5.9764, -8.8104) (5.9911, -8.8243) (6.0059, -8.838) (6.0208, -8.8516) (6.0359, -8.8652) (6.051, -8.8786) (6.0663, -8.892) (6.0817, -8.9052) (6.0972, -8.9184) (6.1128, -8.9315) (6.1285, -8.9445) (6.1444, -8.9574) (6.1603, -8.9702) (6.1764, -8.9829) (6.1926, -8.9956) (6.2089, -9.0081) (6.2252, -9.0206) (6.2417, -9.033) (6.2583, -9.0453) (6.2749, -9.0576) (6.2917, -9.0698) (6.3085, -9.0818) (6.3255, -9.0939) (6.3425, -9.1058) (6.3596, -9.1176) (6.3768, -9.1294) (6.3941, -9.1411) (6.4115, -9.1528) (6.4289, -9.1643) (6.4465, -9.1758) (6.4641, -9.1872) (6.4818, -9.1986) (6.4996, -9.2098) (6.5175, -9.221) (6.5354, -9.2322) (6.5534, -9.2432) (6.5715, -9.2542) (6.5897, -9.2651) (6.6079, -9.276) (6.6263, -9.2868) (6.6447, -9.2975) (6.6631, -9.3081) (6.6817, -9.3187) (6.7003, -9.3292) (6.719, -9.3396) (6.7377, -9.35) (6.7566, -9.3603) (6.7755, -9.3705) (6.7944, -9.3807) (6.8135, -9.3908) (6.8326, -9.4008) (6.8517, -9.4108) (6.871, -9.4207) (6.8903, -9.4305) (6.9096, -9.4403) (6.9291, -9.45) (6.9485, -9.4596) (6.9642, -9.4673) (6.976, -9.473) (6.9838, -9.4768) (6.9877, -9.4787) knots 0 0 0 0 0 0 0.01428571 0.02857143 0.04285714 0.05714286 0.07142857 0.08571429 0.1 0.11428571 0.12857143 0.14285714 0.15714286 0.17142857 0.18571429 0.2 0.21428571 0.22857143 0.24285714 0.25714286 0.27142857 0.28571429 0.3 0.31428571 0.32857143 0.34285714 0.35714286 0.37142857 0.38571429 0.4 0.41428571 0.42857143 0.44285714 0.45714286 0.47142857 0.48571429 0.5 0.51428571 0.52857143 0.54285714 0.55714286 0.57142857 0.58571429 0.6 0.61428571 0.62857143 0.64285714 0.65714286 0.67142857 0.68571429 0.7 0.71428571 0.72857143 0.74285714 0.75714286 0.77142857 0.78571429 0.8 0.81428571 0.82857143 0.84285714 0.85714286 0.87142857 0.88571429 0.9 0.91428571 0.92857143 0.94285714 0.95714286 0.97142857 0.98571429 1 1 1 1 1 1
  arc A74 (6.9877, -9.4787) -> (7.6861, -8.9218) centre (0, 0) ccw
  spline S37 degree 5 poles (7.6861, -8.9218) (7.6851, -8.9175) (7.6832, -8.909) (7.6802, -8.8963) (7.6763, -8.8793) (7.6712, -8.8582) (7.6661, -8.837) (7.6609, -8.816) (7.6556, -8.795) (7.6502, -8.774) (7.6448, -8.7531) (7.6392, -8.7323) (7.6336, -8.7115) (7.6279, -8.6907) (7.6221, -8.67) (7.6163, -8.6494) (7.6104, -8.6288) (7.6043, -8.6082) (7.5982, -8.5878) (7.5921, -8.5673) (7.5858, -8.547) (7.5794, -8.5266) (7.573, -8.5064) (7.5665, -8.4862) (7.5599, -8.466) (7.5532, -8.4459) (7.5464, -8.4259) (7.5396, -8.4059) (7.5326, -8.386) (7.5256, -8.3662) (7.5185, -8.3464) (7.5113, -8.3267) (7.504, -8.307) (7.4966, -8.2874) (7.4891, -8.2679) (7.4816, -8.2484) (7.4739, -8.229) (7.4661, -8.2097) (7.4583, -8.1904) (7.4504, -8.1713) (7.4423, -8.1521) (7.4342, -8.1331) (7.426, -8.1141) (7.4176, -8.0952) (7.4092, -8.0764) (7.4007, -8.0577) (7.3921, -8.039) (7.3833, -8.0204) (7.3745, -8.0019) (7.3656, -7.9835) (7.3565, -7.9652) (7.3474, -7.947) (7.3381, -7.9288) (7.3287, -7.9108) (7.3191, -7.8928) (7.3095, -7.875) (7.2998, -7.8572) (7.2899, -7.8395) (7.28, -7.8219) (7.2699, -7.8044) (7.2597, -7.7871) (7.2492, -7.7699) (7.2386, -7.7529) (7.2278, -7.736) (7.2169, -7.7192) (7.2058, -7.7026) (7.1947, -7.686) (7.1834, -7.6696) (7.172, -7.6532) (7.1604, -7.6371) (7.1484, -7.6213) (7.1384, -7.609) (7.1305, -7.6001) (7.1252, -7.5942) (7.1225, -7.5913) knots -1 -1 -1 -1 -1 -1 -0.98571429 -0.97142857 -0.95714286 -0.94285714 -0.92857143 -0.91428571 -0.9 -0.88571429 -0.87142857 -0.85714286 -0.84285714 -0.82857143 -0.81428571 -0.8 -0.78571429 -0.77142857 -0.75714286 -0.74285714 -0.72857143 -0.71428571 -0.7 -0.68571429 -0.67142857 -0.65714286 -0.64285714 -0.62857143 -0.61428571 -0.6 -0.58571429 -0.57142857 -0.55714286 -0.54285714 -0.52857143 -0.51428571 -0.5 -0.48571429 -0.47142857 -0.45714286 -0.44285714 -0.42857143 -0.41428571 -0.4 -0.38571429 -0.37142857 -0.35714286 -0.34285714 -0.32857143 -0.31428571 -0.3 -0.28571429 -0.27142857 -0.25714286 -0.24285714 -0.22857143 -0.21428571 -0.2 -0.18571429 -0.17142857 -0.15714286 -0.14285714 -0.12857143 -0.11428571 -0.1 -0.08571429 -0.07142857 -0.05714286 -0.04285714 -0.02857143 -0.01428571 0 0 0 0 0 0
  line L37 (7.1225, -7.5913) -> (6.8923, -7.3456)
  arc A75 (6.8936, -6.4965) -> (6.8923, -7.3456) centre (7.3448, -6.9217) ccw
  arc A76 (6.8936, -6.4965) -> (6.9935, -6.3888) centre (0, 0) ccw
  arc A77 (7.8401, -6.3241) -> (6.9935, -6.3888) centre (7.4513, -6.807) ccw
  line L38 (7.8401, -6.3241) -> (8.1024, -6.5353)